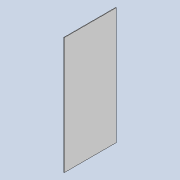
# Autodesk Inventor part: Sponsor and Ad Panel
Saved by Autodesk Inventor 2022 (Build 260153000, 153)
## iProperties
Created: 2023-02-28
Part Number: Sponsor and Ad Panel
Material: Aluminum 6061
Document SubType Name: Modeling
Designer: byrne
Density: 2.7 g/cm^3
Appearance: Aluminum - Flat
Author: byrne
Autodesk Inventor part; units mm, degrees
ref_plane "YZ Plane" through (0, 0, 0) normal (1, 0, 0) x (0, 1, 0)
ref_plane "XZ Plane" through (0, 0, 0) normal (0, 1, 0) x (-1, 0, 0)
ref_plane "XY Plane" through (0, 0, 0) normal (0, 0, 1) x (1, 0, 0)
sketch "Sketch1" plane through (0, 0, 0) normal (1, 0, 0) x (0, 1, 0)
  line L0 (0, 0) -> (1295.4, 0)
  line L1 (1295.4, 0) -> (1295.4, -558.8)
  line L2 (1295.4, -558.8) -> (0, -558.8)
  line L3 (0, -558.8) -> (0, 0)
  dimension "d0" = 1295.4
  dimension "d1" = 558.8
  constraints: 8 end point, 2 parallel, 1 horizontal, 1 perpendicular
  measures "d0" distance of L1.end L2.end
  measures "d1" distance of L0.end L1.end
extrude "Extrusion1" add sketch "Sketch1" along normal blind 3.175
sketch "Sketch2" plane through (3.175, 0, 0) normal (1, 0, 0) x (0, 0, -1)
  line L0 (558.8, 0) -> (558.8, 1295.4) projected
  line L1 (558.8, 1295.4) -> (0, 1295.4) projected
  line L2 (0, 1295.4) -> (0, 0) projected
  line L3 (0, 0) -> (558.8, 0) projected
  circle A0 centre (12.7, 12.7) radius 2.159
  circle A1 centre (546.1, 12.7) radius 2.159
  circle A2 centre (546.1, 1282.7) radius 2.159
  circle A3 centre (12.7, 1282.7) radius 2.159
  dimension "d4" = 4.318
  dimension "d5" = 12.7
  dimension "d6" = 12.7
  dimension "d7" = 4.318
  dimension "d8" = 12.7
  dimension "d9" = 12.7
  dimension "d10" = 4.318
  dimension "d11" = 4.318
  dimension "d12" = 12.7
  dimension "d13" = 12.7
  dimension "d14" = 12.7
  dimension "d15" = 12.7
  constraints: 4 centre point
  measures "d4" diameter of A0
  measures "d5" distance from line of L3 A0.centre
  measures "d6" distance from line of L2 A0.centre
  measures "d7" diameter of A1
  measures "d8" distance from line of L3 A1.centre
  measures "d9" distance from line of L0 A1.centre
  measures "d10" diameter of A2
  measures "d11" diameter of A3
  measures "d12" distance from line of L1 A3.centre
  measures "d13" distance from line of L2 A3.centre
  measures "d14" distance from line of L1 A2.centre
  measures "d15" distance from line of L0 A2.centre
extrude "Extrusion2" cut sketch "Sketch2" against normal blind 3.175 contours A0 | A1 | A2 | A3
equation "\"d9\" = d8"
equation "\"d13\" = d12"
equation "\"d15\" = d14"
body "Solid1"
